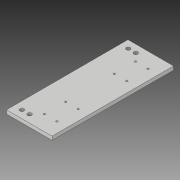
# Autodesk Inventor part: shelf
Saved by Autodesk Inventor 2019 (Build 230136000, 136)
## iProperties
Created: 2019-05-07
Part Number: shelf
Material: Generic
Document SubType Name: Modeling
Designer: devon
Density: 1 g/cm^3
Appearance: Default
Author: devon
Autodesk Inventor part; units mm, degrees
ref_plane "YZ Plane" through (0, 0, 0) normal (1, 0, 0) x (0, 1, 0)
ref_plane "XZ Plane" through (0, 0, 0) normal (0, 1, 0) x (-1, 0, 0)
ref_plane "XY Plane" through (0, 0, 0) normal (0, 0, 1) x (1, 0, 0)
sketch "Sketch1" plane through (0, 0, 0) normal (0, 1, 0) x (-1, 0, 0)
  line L0 (-37.5, 100) -> (37.5, 100)
  line L1 (37.5, 100) -> (37.5, -100)
  line L2 (37.5, -100) -> (-37.5, -100)
  line L3 (-37.5, -100) -> (-37.5, 100)
  line L4 (-37.5, 100) -> (37.5, -100) construction
  line L5 (37.5, 100) -> (-37.5, -100) construction
  point P0 (0, 0)
  dimension "d0" = 200
  dimension "d1" = 75
  constraints: 12 end point, 2 midpoint, 2 parallel, 1 horizontal, 1 perpendicular
  measures "d0" distance of L0.end L1.end
  measures "d1" distance of L0.start L0.end
extrude "Extrusion1" add sketch "Sketch1" along normal blind 6
sketch "Sketch2" plane through (0, 6, 0) normal (0, 1, 0) x (1, 0, 0)
  circle A0 centre (-24.5, -87.5) radius 3.25
  circle A1 centre (-12, -87.5) radius 3.25
  circle A2 centre (-24.5, 87.5) radius 3.25
  circle A3 centre (-12, 87.5) radius 3.25
  line L0 (-37.5, 100) -> (-37.5, -100) projected
  line L1 (-37.5, -100) -> (37.5, -100) projected
  line L2 (37.5, 100) -> (-37.5, 100) projected
  point P0 (0, 0)
  dimension "d4" = 6.5
  dimension "d5" = 6.5
  dimension "d6" = 12.5
  dimension "d7" = 13
  dimension "d8" = 12.5
  dimension "d9" = 12.5
  dimension "d10" = 6.5
  dimension "d11" = 6.5
  dimension "d12" = 12.5
  dimension "d13" = 13
  dimension "d14" = 12.5
  dimension "d15" = 12.5
  constraints: 4 centre point
  measures "d4" diameter of A0
  measures "d5" diameter of A1
  measures "d6" distance of A1.centre A0.centre
  measures "d7" distance from line of L0 A0.centre
  measures "d8" distance from line of L1 A0.centre
  measures "d9" distance from line of L1 A1.centre
  measures "d10" diameter of A2
  measures "d11" diameter of A3
  measures "d12" distance of A3.centre A2.centre
  measures "d13" distance from line of L0 A2.centre
  measures "d14" distance from line of L2 A2.centre
  measures "d15" distance from line of L2 A3.centre
extrude "Extrusion2" cut sketch "Sketch2" against normal through all
sketch "Sketch3" plane through (0, 6, 0) normal (0, 1, 0) x (1, 0, 0)
  circle A0 centre (0, -75.052) radius 1.45
  circle A1 centre (20.574, -75.052) radius 1.45
  circle A2 centre (0, -40) radius 1.45
  circle A3 centre (20.574, -40) radius 1.45
  circle A4 centre (0, 40) radius 1.45
  circle A5 centre (20.574, 40) radius 1.45
  circle A6 centre (0, 75.052) radius 1.45
  circle A7 centre (20.574, 75.052) radius 1.45
  point P0 (0, 0)
  dimension "d18" = 2.9
  dimension "d19" = 2.9
  dimension "d20" = 2.9
  dimension "d21" = 2.9
  dimension "d22" = 20.574
  dimension "d23" = 35.052
  dimension "d24" = 35.052
  dimension "d25" = 20.574
  dimension "d26" = 0
  dimension "d27" = 40
  dimension "d28" = 2.9
  dimension "d29" = 2.9
  dimension "d30" = 2.9
  dimension "d31" = 2.9
  dimension "d32" = 20.574
  dimension "d33" = 35.052
  dimension "d34" = 35.052
  dimension "d35" = 20.574
  dimension "d36" = 0
  dimension "d37" = 0
  dimension "d38" = 40
  dimension "d39" = 40
  dimension "d42" = 0
  dimension "d43" = 40
  constraints: 8 centre point
  measures "d18" diameter of A0
  measures "d19" diameter of A2
  measures "d20" diameter of A3
  measures "d21" diameter of A1
  measures "d22" distance of A1.centre A0.centre
  measures "d23" distance of A2.centre A0.centre
  measures "d24" distance of A1.centre A3.centre
  measures "d25" distance of A3.centre A2.centre
  measures "d26" horizontal distance of point (0, 0) A0.centre
  measures "d27" distance of point (0, 0) A2.centre
  measures "d28" diameter of A4
  measures "d29" diameter of A6
  measures "d30" diameter of A7
  measures "d31" diameter of A5
  measures "d32" distance of A5.centre A4.centre
  measures "d33" distance of A6.centre A4.centre
  measures "d34" distance of A5.centre A7.centre
  measures "d35" distance of A7.centre A6.centre
  measures "d36" horizontal distance of point (0, 0) A4.centre
  measures "d37" horizontal distance of point (0, 0) A6.centre
  measures "d38" distance of point (0, 0) A4.centre
  measures "d39" vertical distance of point (0, 0) A5.centre
  measures "d42" horizontal distance of point (0, 0) A2.centre
  measures "d43" vertical distance of point (0, 0) A3.centre
extrude "Extrusion3" cut sketch "Sketch3" against normal through all
body "Solid1"
